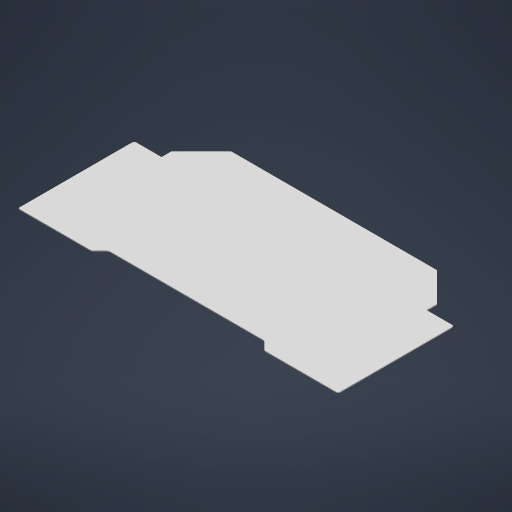
# Autodesk Inventor part: base_plate_isolation
Saved by Autodesk Inventor 2024 (Build 280153000, 153)
## iProperties
Created: 2024-03-21
Part Number: base_plate_isolation
Material: Všeobecné
Document SubType Name: Modeling
Designer: Simak
Density: 1 g/cm^3
Appearance: Výchozí
Author: Simak
Autodesk Inventor part; units mm, degrees
ref_plane "YZ Plane" through (0, 0, 0) normal (1, 0, 0) x (0, 1, 0)
ref_plane "XZ Plane" through (0, 0, 0) normal (0, 1, 0) x (-1, 0, 0)
ref_plane "XY Plane" through (0, 0, 0) normal (0, 0, 1) x (1, 0, 0)
sketch "Náčrt1" plane through (0, 0, 0) normal (0, 1, 0) x (-1, 0, 0)
  line L0 (24, -47.25) -> (19.6818, -47.25)
  line L1 (24, -47.25) -> (24, -17.0868)
  line L2 (24, -17.0868) -> (49.75, -17.0868)
  line L3 (49.75, 48.4103) -> (49.75, -17.0868)
  line L4 (49.75, 48.4103) -> (-49.75, 48.4103)
  line L5 (-49.75, 48.4103) -> (-49.75, -17.0868)
  line L6 (-24, -17.0868) -> (-49.75, -17.0868)
  line L7 (-24, -47.25) -> (-24, -17.0868)
  line L8 (-19.6818, -47.25) -> (-24, -47.25)
  arc A0 (-18.3182, -47.25) -> (-19.6818, -47.25) centre (-19, -43.5625) ccw
  line L9 (-12, -47.25) -> (-18.3182, -47.25)
  line L10 (-12, -47.25) -> (-12, -40)
  line L11 (-12, -40) -> (-3.25, -40)
  arc A1 (-3, -40.25) -> (-3.25, -40) centre (-3.25, -40.25) ccw
  line L12 (-3, -40.25) -> (-3, -40.6521)
  arc A2 (-3, -40.6521) -> (-2.6294, -40.8711) centre (-2.75, -40.6521) ccw
  arc A3 (2.0811, -47.25) -> (-2.6294, -40.8711) centre (-0.7, -44.375) ccw
  line L13 (18.3182, -47.25) -> (2.0811, -47.25)
  arc A4 (19.6818, -47.25) -> (18.3182, -47.25) centre (19, -43.5625) ccw
  arc A5 (-30.6049, -8.4571) -> (-29.8978, -8.75) centre (-29.8978, -7.75) ccw
  line L14 (-30.6049, -8.4571) -> (-39.25, 0.188)
  line L15 (-39.25, 2.8608) -> (-39.25, 0.188)
  line L16 (-46.25, 2.8608) -> (-39.25, 2.8608)
  ellipse E0 centre (-46.25, 4.3321) end of major axis (-46.25, 2.8608) minor radius 1 (-47.25, 4.3321) -> (-46.25, 2.8608) ccw
  line L17 (-47.25, 4.3321) -> (-47.25, 36.8221)
  arc A6 (-46.25, 37.8221) -> (-47.25, 36.8221) centre (-46.25, 36.8221) ccw
  line L18 (-46.25, 37.8221) -> (-45.25, 37.8221)
  arc A7 (-45.25, 37.8221) -> (-44.25, 38.8221) centre (-45.25, 38.8221) ccw
  line L19 (-44.25, 41.8041) -> (-44.25, 38.8221)
  arc A8 (-36.75, 41.8041) -> (-44.25, 41.8041) centre (-40.5, 41.8041) ccw
  line L20 (-36.75, 38.8221) -> (-36.75, 41.8041)
  arc A9 (-36.75, 38.8221) -> (-35.75, 37.8221) centre (-35.75, 38.8221) ccw
  line L21 (-35.75, 37.8221) -> (-25.4142, 37.8221)
  arc A10 (-24.7071, 37.5292) -> (-25.4142, 37.8221) centre (-25.4142, 36.8221) ccw
  line L22 (-22.7929, 35.615) -> (-24.7071, 37.5292)
  arc A11 (-22.7929, 35.615) -> (-22.0858, 35.3221) centre (-22.0858, 36.3221) ccw
  line L23 (-22.0858, 35.3221) -> (22.0858, 35.3221)
  arc A12 (22.0858, 35.3221) -> (22.7929, 35.615) centre (22.0858, 36.3221) ccw
  line L24 (22.7929, 35.615) -> (24.7071, 37.5292)
  arc A13 (25.4142, 37.8221) -> (24.7071, 37.5292) centre (25.4142, 36.8221) ccw
  line L25 (35.75, 37.8221) -> (25.4142, 37.8221)
  arc A14 (35.75, 37.8221) -> (36.75, 38.8221) centre (35.75, 38.8221) ccw
  line L26 (36.75, 38.8221) -> (36.75, 41.8041)
  arc A15 (44.25, 41.8041) -> (36.75, 41.8041) centre (40.5, 41.8041) ccw
  line L27 (44.25, 41.8041) -> (44.25, 38.8221)
  arc A16 (44.25, 38.8221) -> (45.25, 37.8221) centre (45.25, 38.8221) ccw
  line L28 (46.25, 37.8221) -> (45.25, 37.8221)
  arc A17 (47.25, 36.8221) -> (46.25, 37.8221) centre (46.25, 36.8221) ccw
  line L29 (47.25, 4.3321) -> (47.25, 36.8221)
  ellipse E1 centre (46.25, 4.3321) end of major axis (46.25, 2.8608) minor radius 1 (46.25, 2.8608) -> (47.25, 4.3321) ccw
  line L30 (46.25, 2.8608) -> (39.25, 2.8608)
  line L31 (39.25, 2.8608) -> (39.25, 0.188)
  line L32 (30.6049, -8.4571) -> (39.25, 0.188)
  arc A18 (29.8978, -8.75) -> (30.6049, -8.4571) centre (29.8978, -7.75) ccw
  line L33 (29.8978, -8.75) -> (-29.8978, -8.75)
  line L34 (-3.45, -32.125) -> (-3.45, -26.625)
  line L35 (-3.45, -26.625) -> (2.05, -26.625)
  line L36 (2.05, -26.625) -> (2.05, -32.125)
  line L37 (2.05, -32.125) -> (-3.45, -32.125)
  line L38 (6.3401, -40.3942) -> (9.6599, -40.3942)
  line L39 (9.6599, -40.3942) -> (11.3198, -43.2692)
  line L40 (11.3198, -43.2692) -> (9.6599, -46.1442)
  line L41 (9.6599, -46.1442) -> (6.3401, -46.1442)
  line L42 (6.3401, -46.1442) -> (4.6802, -43.2692)
  line L43 (4.6802, -43.2692) -> (6.3401, -40.3942)
  circle A19 centre (-19, -22.9375) radius 1.75
  circle A20 centre (-20, 39.763) radius 1.75
  circle A21 centre (20, 39.763) radius 1.75
  circle A22 centre (19, -22.9375) radius 1.75
  circle A23 centre (42.25, -8.75) radius 1.75
  circle A24 centre (-42.25, -8.75) radius 1.75
  line L44 (38.75, 0.3951) -> (38.75, 3.3608)
  line L45 (38.75, 3.3608) -> (46.25, 3.3608)
  line L46 (46.75, 4.3321) -> (46.75, 36.8221)
  arc A25 (46.75, 36.8221) -> (46.25, 37.3221) centre (46.25, 36.8221) ccw
  line L47 (46.25, 37.3221) -> (45.25, 37.3221)
  arc A26 (43.75, 38.8221) -> (45.25, 37.3221) centre (45.25, 38.8221) ccw
  line L48 (43.75, 38.8221) -> (43.75, 41.8041)
  arc A27 (43.75, 41.8041) -> (37.25, 41.8041) centre (40.5, 41.8041) ccw
  line L49 (37.25, 41.8041) -> (37.25, 38.8221)
  arc A28 (35.75, 37.3221) -> (37.25, 38.8221) centre (35.75, 38.8221) ccw
  line L50 (35.75, 37.3221) -> (25.4142, 37.3221)
  arc A29 (25.4142, 37.3221) -> (25.0607, 37.1756) centre (25.4142, 36.8221) ccw
  line L51 (25.0607, 37.1756) -> (23.1464, 35.2614)
  arc A30 (22.0858, 34.8221) -> (23.1464, 35.2614) centre (22.0858, 36.3221) ccw
  line L52 (22.0858, 34.8221) -> (-22.0858, 34.8221)
  arc A31 (-23.1464, 35.2614) -> (-22.0858, 34.8221) centre (-22.0858, 36.3221) ccw
  line L53 (-23.1464, 35.2614) -> (-25.0607, 37.1756)
  arc A32 (-25.0607, 37.1756) -> (-25.4142, 37.3221) centre (-25.4142, 36.8221) ccw
  line L54 (-25.4142, 37.3221) -> (-35.75, 37.3221)
  arc A33 (-37.25, 38.8221) -> (-35.75, 37.3221) centre (-35.75, 38.8221) ccw
  line L55 (-37.25, 38.8221) -> (-37.25, 41.8041)
  arc A34 (-37.25, 41.8041) -> (-43.75, 41.8041) centre (-40.5, 41.8041) ccw
  line L56 (-43.75, 41.8041) -> (-43.75, 38.8221)
  arc A35 (-45.25, 37.3221) -> (-43.75, 38.8221) centre (-45.25, 38.8221) ccw
  line L57 (-45.25, 37.3221) -> (-46.25, 37.3221)
  arc A36 (-46.25, 37.3221) -> (-46.75, 36.8221) centre (-46.25, 36.8221) ccw
  line L58 (-46.75, 36.8221) -> (-46.75, 4.3321)
  line L59 (-46.25, 3.3608) -> (-38.75, 3.3608)
  line L60 (-38.75, 3.3608) -> (-38.75, 0.3951)
  line L61 (-38.75, 0.3951) -> (-30.2513, -8.1036)
  arc A37 (-30.2513, -8.1036) -> (-29.8978, -8.25) centre (-29.8978, -7.75) ccw
  line L62 (-29.8978, -8.25) -> (29.8978, -8.25)
  arc A38 (29.8978, -8.25) -> (30.2513, -8.1036) centre (29.8978, -7.75) ccw
  line L63 (30.2513, -8.1036) -> (38.75, 0.3951)
  line L64 (45.25, 37.3221) -> (35.75, 37.3221)
  line L65 (-35.75, 37.3221) -> (-45.25, 37.3221)
  spline S0 degree 5 poles (46.25, 3.3609) (46.281, 3.3609) (46.3118, 3.3675) (46.3409, 3.3802) (46.4606, 3.4487) (46.5476, 3.5625) (46.6014, 3.6535) (46.6833, 3.8417) (46.7286, 4.0407) (46.7429, 4.1374) (46.75, 4.2348) (46.75, 4.3321) knots 0 0 0 0 0 0 0.13219 0.13219 0.13219 0.585181 0.585181 0.585181 1 1 1 1 1 1
  spline S1 degree 5 poles (-46.75, 4.3321) (-46.75, 4.2348) (-46.7429, 4.1374) (-46.7286, 4.0407) (-46.6833, 3.8417) (-46.6014, 3.6535) (-46.5476, 3.5625) (-46.4606, 3.4487) (-46.3409, 3.3802) (-46.3118, 3.3675) (-46.281, 3.3609) (-46.25, 3.3609) knots 0 0 0 0 0 0 0.414819 0.414819 0.414819 0.86781 0.86781 0.86781 1 1 1 1 1 1
  point P0 (0, 0)
  point P1 (0, 0)
  dimension "d0" = 0.5
  constraints: 132 end point, 66 point on circle, 39 centre point, 4 parallel, 2 collinear, 1 tangent, 45 other
  measures "d0" distance between parallel lines of L32 L63
extrude "Vysunutí1" add sketch "Náčrt1" along normal blind 0.2 contours L63 A38 L62 A37 L61 L60 L59 S1 L58 A36 L57 L65 L54 A32 L53 A31 L52 A30 L51 A29 L50 L64 L47 A25 L46 S0 L45 L44
